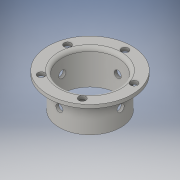
# Autodesk Inventor part: Pipe Mounting Sleeve_2
Saved by Autodesk Inventor 2016 (Build 200138000, 138)
## iProperties
Created: 2016-03-16
Part Number: Pipe Mounting Sleeve_2
Material: Generic
Document SubType Name: Modeling
Designer: v40-4
Density: 1 g/cm^3
Appearance: Default
Author: v40-4
## iProperties of the stored document Pipe Mounting Sleeve_3DPrint.ipt
Created: 2016-03-17
Part Number: Pipe Mounting Sleeve_3DPrint
Material: Generic
Document SubType Name: Modeling
Designer: noory
Density: 1 g/cm^3
Appearance: Default
Author: noory
Autodesk Inventor part; units mm, degrees
ref_plane "YZ Plane" through (0, 0, 0) normal (1, 0, 0) x (0, 1, 0)
ref_plane "XZ Plane" through (0, 0, 0) normal (0, 1, 0) x (-1, 0, 0)
sketch "Sketch1" plane through (0, 0, 0) normal (0, 1, 0) x (-1, 0, 0)
  circle A0 centre (0, 0) radius 25.4
  dimension "d0" = 50.8
  constraints: 1 centre point, 1 coincident
  measures "d0" diameter of A0
extrude "Extrusion1" add sketch "Sketch1" along normal blind 25.4
shell "Shell1" thickness 2.54 outward yes removed faces 1 at (7.2508, 0, -1.9085)
sketch "Sketch2" plane through (0, 27.94, 0) normal (0, 1, 0) x (1, 0, 0)
  circle A0 centre (0, 0) radius 38.1
  dimension "d4" = 76.2
  constraints: 1 centre point, 1 coincident
  measures "d4" diameter of A0
extrude "Extrusion2" add sketch "Sketch2" along normal blind 3.175
sketch "Sketch3" plane through (0, 25.4, 0) normal (0, -1, 0) x (1, 0, 0)
  circle A0 centre (0, 0) radius 25.4 projected
extrude "Extrusion3" cut sketch "Sketch3" against normal up to surface (5.715 mm away)
sketch "Sketch4" plane through (0, 31.115, 0) normal (0, 1, 0) x (1, 0, 0)
  circle A0 centre (0, 0) radius 25.4 projected
  circle A1 centre (0, 0) radius 38.1 projected
  line L0 (0, 53.34) -> (0, -53.34) projected
  circle A2 centre (0, 0) radius 31.75 construction
  point P0 (0, 31.75)
  dimension "d9" = 63.5
  constraints: 1 coincident, 1 point on line, 1 vertical alignment, 2 other
hole "Hole1" at (0, 31.115, -31.75) direction (0, -1, 0) diameter 6.477 end through all
pattern_circular "Circular Pattern1" count 5 over 360 about axis through (0, 0, 0) along (0, 1, 0) of "Hole1"
fillet "Fillet1" radius 3.175 1 edges at (-25.4, 31.115, 0)
ref_plane "Work Plane1" through (0, 15.24, 0) normal (0, 1, 0) x (1, 0, 0)
sketch "Sketch5" plane through (0, 15.24, 0) normal (0, 1, 0) x (1, 0, 0)
  circle A0 centre (0, 0) radius 25.4 projected
  line L0 (0, 53.34) -> (0, -53.34) projected
  point P0 (0, 25.4)
  constraints: 1 point on line, 1 vertical alignment, 1 other
sketch "Sketch6" plane through (0, 0, 0) normal (0, 0, 1) x (1, 0, 0)
  line L0 (-53.34, 15.24) -> (53.34, 15.24) projected
  point P0 (0, 0)
  point P1 (0, 15.24)
  constraints: 1 midpoint
hole "Hole2" at (0, 15.24, 0) direction (0, 0, -1) diameter 6.477 end through all
pattern_circular "Circular Pattern2" count 4 over 360 about axis through (0, 0, 0) along (0, 1, 0) of "Hole2"
body "Solid1"
